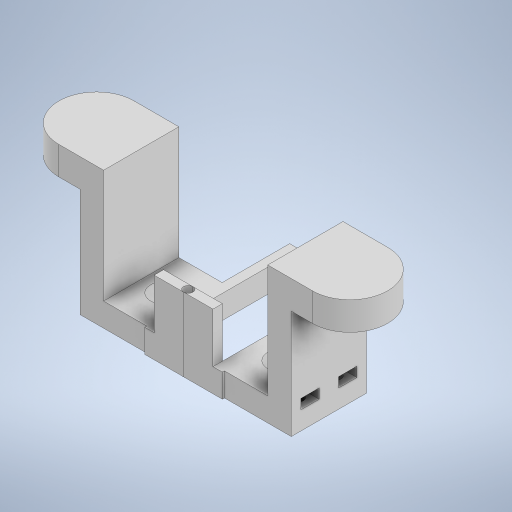
# Autodesk Inventor part: Basis of steering
Saved by Autodesk Inventor 2023 (Build 270158000, 158)
## iProperties
Created: 2023-05-17
Part Number: Basis of steering
Material: Типовые
Document SubType Name: Modeling
Designer: ivanc
Density: 1 g/cm^3
Appearance: По умолчанию
Author: ivanc
Autodesk Inventor part; units mm, degrees
ref_plane "YZ Plane" through (0, 0, 0) normal (1, 0, 0) x (0, 1, 0)
ref_plane "XZ Plane" through (0, 0, 0) normal (0, 1, 0) x (-1, 0, 0)
ref_plane "XY Plane" through (0, 0, 0) normal (0, 0, 1) x (1, 0, 0)
sketch "Эскиз1" plane through (0, 0, 0) normal (0, 1, 0) x (-1, 0, 0)
  line L0 (-8.725, 8) -> (8.725, 8)
  line L1 (8.725, 8) -> (8.725, -8)
  line L2 (8.725, -8) -> (-8.725, -8)
  line L3 (-8.725, -8) -> (-8.725, 8)
  line L4 (-8.725, 8) -> (8.725, -8) construction
  line L5 (8.725, 8) -> (-8.725, -8) construction
  point P0 (0, 0)
  dimension "d0" = 17.45
  dimension "d1" = 16
  constraints: 12 end point, 2 midpoint, 2 parallel, 1 horizontal, 1 perpendicular
  measures "d0" distance of L1.end L2.end
  measures "d1" distance of L0.end L1.end
extrude "Выдавливание1" add sketch "Эскиз1" along normal blind 5
sketch "Эскиз2" plane through (-8.725, 0, -8) normal (-1, 0, 0) x (0, 0, 1)
  line L0 (0, 23.1) -> (16, 23.1)
  line L1 (16, 23.1) -> (16, 0)
  line L2 (16, 0) -> (0, 0)
  line L3 (0, 0) -> (0, 23.1)
  line L4 (16, 0) -> (16, 5) projected
  line L5 (0, 0) -> (0, 5) projected
  line L6 (0, 0) -> (16, 0) projected
  line L7 (0, 5) -> (16, 5) projected
  point P0 (8, 0)
  dimension "d5" = 18.1
  constraints: 8 end point, 3 collinear, 2 parallel, 1 horizontal, 1 perpendicular
  measures "d5" distance between parallel lines of L7 L0
extrude "Выдавливание2" add sketch "Эскиз2" along normal blind 5
sketch "Эскиз3" plane through (-8.725, 23.1, 8) normal (0, 1, 0) x (1, 0, 0)
  line L0 (0, 16) -> (-17.5, 16)
  line L1 (-17.5, 16) -> (-17.5, 0)
  line L2 (-17.5, 0) -> (0, 0)
  line L3 (0, 0) -> (0, 16)
  line L4 (0, 0) -> (-5, 0) projected
  circle A0 centre (-9.5, 8) radius 8
  line L5 (-5, 0) -> (-5, 16) projected
  point P0 (-9.5, 16)
  point P1 (-9.5, 0)
  point P2 (-5, 8)
  dimension "d49" = 4.5
  constraints: 8 end point, 3 tangent, 2 parallel, 1 centre point, 1 collinear, 1 horizontal, 1 midpoint, 1 perpendicular
  measures "d49" distance of point (-5, 8) A0.centre
extrude "Выдавливание3" add sketch "Эскиз3" along normal blind 6 contours L3 L2 L5 A0 L0 | L5 A0 L0 | A0 L5 | A0 L5 | L2 A0 L5
sketch "Эскиз7" plane through (0, 0, 0) normal (0, -1, 0) x (1, 0, 0)
  line L0 (-8.725, -8) -> (-8.725, 8) construction
  line L1 (-8.725, 8) -> (-8.725, -8) construction
  line L2 (-13.725, 8) -> (-13.725, -8) construction
  line L3 (-8.725, -8) -> (-13.725, -8) construction
  line L4 (-13.725, -8) -> (-13.725, 8) construction
  line L5 (-13.725, 8) -> (-8.725, 8) construction
  line L6 (-8.725, 8) -> (-8.725, -8) construction
  line L7 (-13.725, -8) -> (-13.725, 8) projected
  line L8 (-13.725, 0) -> (-8.725, 0) construction
  line L9 (-11.225, -4) -> (-11.225, 4)
  point P0 (0, 0)
  point P1 (-11.225, 0)
  dimension "d34" = 8
  constraints: 12 end point, 4 midpoint, 2 parallel, 1 horizontal, 1 perpendicular, 1 vertical
  measures "d34" distance of L9.start L9.end
hole "Отверстие3" at (-11.225, 0, -4) at (-11.225, 0, 4) direction (0, 1, 0) diameter 2.2 depth 6
sketch "Эскиз8" plane through (0, 0, 0) normal (0, -1, 0) x (1, 0, 0)
  circle A0 centre (-11.225, -4) radius 1.1 projected
  line L0 (-13.4767, -4) -> (-12.3508, -2.05) construction
  line L1 (-12.3508, -2.05) -> (-10.0992, -2.05)
  line L2 (-10.0992, -2.05) -> (-8.9733, -4)
  line L3 (-8.9733, -4) -> (-10.0992, -5.95)
  line L4 (-10.0992, -5.95) -> (-12.3508, -5.95)
  line L5 (-12.3508, -5.95) -> (-13.4767, -4) construction
  circle A1 centre (-11.225, 4) radius 1.1 projected
  line L6 (-13.4767, 4) -> (-12.3508, 5.95) construction
  line L7 (-12.3508, 5.95) -> (-10.0992, 5.95)
  line L8 (-10.0992, 5.95) -> (-8.9733, 4)
  line L9 (-8.9733, 4) -> (-10.0992, 2.05)
  line L10 (-10.0992, 2.05) -> (-12.3508, 2.05)
  line L11 (-12.3508, 2.05) -> (-13.4767, 4) construction
  line L12 (-13.725, -8) -> (-13.725, 8) projected
  line L13 (-12.3508, -5.95) -> (-13.725, -5.95)
  line L14 (-13.725, -5.95) -> (-13.725, -2.05)
  line L15 (-13.725, -2.05) -> (-12.3508, -2.05)
  line L16 (-12.3508, -2.05) -> (-12.3508, -5.95) construction
  line L17 (-12.3508, 2.05) -> (-13.725, 2.05)
  line L18 (-13.725, 2.05) -> (-13.725, 5.95)
  line L19 (-13.725, 5.95) -> (-12.3508, 5.95)
  line L20 (-12.3508, 5.95) -> (-12.3508, 2.05) construction
  point P0 (0, 0)
  dimension "d42" = 3.9
  constraints: 40 end point, 5 parallel, 4 collinear, 4 perpendicular, 2 coincident, 2 horizontal, 26 other
  measures "d42" distance between parallel lines of L1 L4
extrude "Выдавливание5" cut sketch "Эскиз8" along normal blind 2.1 from surface at -6
sketch "Эскиз4" plane through (-8.725, 23.1, 8) normal (0, -1, 0) x (1, 0, 0)
  arc A0 (-9.5, 0) -> (-9.5, -16) centre (-9.5, -8) ccw projected
  circle A1 centre (-12.5, -8) radius 4
  arc A2 (-9.5, 0) -> (-9.5, -16) centre (-9.5, -8) ccw projected
  line L0 (-17.5, -8) -> (-16.5, -8) construction
  line L1 (-16.5, -8) -> (-9.5, -8) construction
  point P0 (8.725, -8)
  dimension "d45" = 8
  dimension "d46" = 1
  constraints: 4 end point, 2 horizontal, 2 point on circle, 1 horizontal alignment, 1 point on line, 2 other
  measures "d46" distance of L0.start L0.end
extrude "Выдавливание6" cut sketch "Эскиз4" against normal blind 3
sketch "Эскиз5" plane through (0, 5, 0) normal (0, 1, 0) x (1, 0, 0)
  line L0 (-8.725, 8) -> (-8.725, -8) projected
  line L1 (-8.725, 0) -> (-3.725, 0) construction
  point P0 (0, 0)
  dimension "d22" = 5
  constraints: 2 end point, 1 horizontal, 1 midpoint
  measures "d22" distance of L1.start L1.end
hole "Отверстие2" at (-3.725, 5, 0) direction (0, -1, 0) diameter 3.2 end through all countersink diameter 6 countersink angle 90
mirror "Зеркальное отражение1" about plane through (8.725, 0, 8) normal (1, 0, 0)
sketch "Эскиз9" plane through (0, 0, 0) normal (0, -1, 0) x (1, 0, 0)
  line L0 (-8.725, 8) -> (26.175, 8) construction
  line L1 (8.725, 8) -> (8.725, -8) construction
  line L2 (-8.725, -8) -> (26.175, -8) construction
  line L3 (2.475, -16.35) -> (14.975, -16.35) construction
  line L4 (14.975, -16.35) -> (14.975, 6.45) construction
  line L5 (14.975, 6.45) -> (2.475, 6.45) construction
  line L6 (2.475, 6.45) -> (2.475, -16.35) construction
  line L7 (2.475, -16.35) -> (14.975, 6.45) construction
  line L8 (14.975, -16.35) -> (2.475, 6.45) construction
  line L9 (16.975, 8.45) -> (0.475, 8.45)
  line L10 (0.475, 8.45) -> (0.475, -22.35)
  line L11 (0.475, -22.35) -> (16.975, -22.35)
  line L12 (16.975, -22.35) -> (16.975, 8.45)
  point P0 (0, 0)
  point P1 (8.725, -4.95)
  point P2 (8.725, 0)
  dimension "d50" = 12.5
  dimension "d51" = 22.8
  dimension "d59" = 4.95
  dimension "d68" = 6
  dimension "d69" = 2
  dimension "d70" = 2
  dimension "d71" = 2
  constraints: 22 end point, 5 midpoint, 4 parallel, 2 horizontal, 2 perpendicular, 1 point on line
  measures "d50" distance of L5.end L4.end
  measures "d51" distance of L4.end L3.end
  measures "d59" distance of point (8.725, 0) point (8.725, -4.95)
  measures "d68" distance between parallel lines of L3 L11
  measures "d69" distance between parallel lines of L5 L9
  measures "d70" distance between parallel lines of L12 L4
  measures "d71" distance between parallel lines of L6 L10
extrude "Выдавливание7" add sketch "Эскиз9" against normal up to surface (5 mm away)
sketch "Эскиз10" plane through (0, 5, 0) normal (0, 1, 0) x (1, 0, 0)
  line L0 (2.475, -6.45) -> (14.975, -6.45)
  line L1 (14.975, -6.45) -> (14.975, 16.35)
  line L2 (14.975, 16.35) -> (2.475, 16.35)
  line L3 (2.475, 16.35) -> (2.475, -6.45)
  line L4 (2.475, -6.45) -> (14.975, 16.35) construction
  line L5 (14.975, -6.45) -> (2.475, 16.35) construction
  line L6 (-8.725, 8) -> (0.475, 8) projected
  line L7 (16.975, -8) -> (0.475, 8) construction
  line L8 (16.975, 8) -> (26.175, 8) projected
  line L9 (-8.725, -8) -> (0.475, -8) projected
  line L10 (16.975, 8) -> (0.475, -8) construction
  line L11 (16.975, -8) -> (26.175, -8) projected
  line L12 (8.725, 0) -> (8.725, 4.95)
  point P0 (0, 0)
  dimension "d54" = 12.5
  dimension "d55" = 22.8
  dimension "d72" = 4.95
  constraints: 18 end point, 3 midpoint, 2 parallel, 1 horizontal, 1 perpendicular, 1 vertical
  measures "d54" distance of L2.end L1.end
  measures "d55" distance of L1.end L0.end
  measures "d72" distance of L12.start L12.end
extrude "Выдавливание8" cut sketch "Эскиз10" against normal through all
sketch "Эскиз11" plane through (0, 0, 0) normal (0, -1, 0) x (1, 0, 0)
  line L0 (8.725, -22.35) -> (8.725, -16.35) construction
  line L1 (12.725, -19.35) -> (4.725, -19.35)
  line L2 (14.975, -16.35) -> (2.475, -16.35) projected
  line L3 (0.475, -22.35) -> (16.975, -22.35) projected
  point P0 (0, 0)
  point P1 (8.725, -19.35)
  dimension "d60" = 8
  constraints: 4 end point, 4 midpoint, 1 horizontal
  measures "d60" distance of L1.start L1.end
hole "Отверстие4" at (12.725, 0, -19.35) at (4.725, 0, -19.35) direction (0, 1, 0) diameter 2.2 end through all countersink diameter 4.2 countersink angle 90
sketch "Эскиз12" plane through (0, 5, 0) normal (0, 1, 0) x (1, 0, 0)
  line L0 (2.475, -6.45) -> (14.975, -6.45) projected
  line L1 (14.975, -6.45) -> (2.475, -6.45)
  line L2 (2.475, -6.45) -> (2.475, -8.45)
  line L3 (2.475, -8.45) -> (14.975, -8.45)
  line L4 (14.975, -8.45) -> (14.975, -6.45)
  line L5 (16.975, -8.45) -> (0.475, -8.45) projected
  point P0 (0, 0)
  constraints: 8 end point, 2 parallel, 1 collinear, 1 horizontal, 1 perpendicular
extrude "Выдавливание9" add sketch "Эскиз12" along normal blind 10.6
sketch "Эскиз13" plane through (0, 15.6, 0) normal (0, 1, 0) x (1, 0, 0)
  line L0 (16.975, -8.45) -> (0.475, -8.45) projected
  line L1 (8.725, -8.45) -> (8.725, -6.45) construction
  line L2 (2.475, -6.45) -> (14.975, -6.45) projected
  point P0 (0, 0)
  point P1 (8.725, -7.45)
  constraints: 3 midpoint, 2 end point
hole "Отверстие5" at (8.725, 15.6, 7.45) direction (0, -1, 0) diameter 2 depth 6000 tip angle 118
